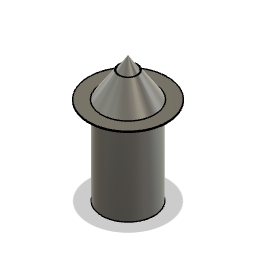
Shielding for CAMECA electrodes v1 (Autodesk Fusion 360 design; units mm, degrees)
Autodesk Fusion 360 part; units mm, degrees
sketch "Sketch1" plane through (0, 0, 0) normal (0, 0, 1) x (1, 0, 0)
  line L0 (0, 3) -> (1, 3) construction
  line L1 (0, 0) -> (3, 0) construction
  line L2 (1, 3) -> (3, 0)
  line L3 (3, 0) -> (4.5, 0)
  line L4 (4.5, 0) -> (4.5, 0.1)
  line L5 (1, 3) -> (1.0832, 3.0555)
  line L6 (4.5, 0.1) -> (3.0535, 0.1)
  line L7 (3.0535, 0.1) -> (1.0832, 3.0555)
  line L8 (0, 4.5) -> (3, 0)
  line L9 (3, 0) -> (3, -10)
  line L10 (3, -10) -> (0, -10)
  line L11 (0, 1.75) -> (0, 22.5)
  line L12 (0, 4.5) -> (0, -10)
  dimension "d1" = 1
  dimension "d3" = 3
  dimension "d4" = 3
  dimension "d5" = 1.5
  dimension "d6" = 0.1
  dimension "d7" = 0.1
  dimension "d9" = 123.69
  dimension "d11" = 10
  constraint horizontal L0
  constraint coincident L1.start origin
  constraint horizontal L1
  constraint parallel L1 L3
  constraint perpendicular L3 L4
  constraint perpendicular L2 L5
  constraint perpendicular L4 L6
  constraint parallel L2 L7
  constraint parallel L2 L8
  constraint vertical L9
  constraint perpendicular L9 L10
  constraint coincident L8.start L11
  constraint perpendicular L10 L12
  measures "d1" distance of L0.start L0.end
  measures "d3" distance of L1.start L1.end
  measures "d4" distance of L1.start L0.start
  measures "d5" distance of L1.end L3.end
  measures "d6" distance of L3.end L4.end
  measures "d7" distance of L0.end L5.end
  measures "d9" angle of L6 L7
  measures "d11" distance of L1.end L9.end
revolve "Revolve1" add sketch "Sketch1" angle 360 about axis through (0, 1.75, 0) along (0, 1, 0) contours L2 L3 L4 L5 L6 L7 L8 makes body 1
revolve "Revolve2" add sketch "Sketch1" angle 360 about axis through (0, 1.75, 0) along (0, 1, 0) separate body contours L2 L8 L9 L10 L11 L12 makes body 2
named bodies: "Shielding", "Shielding Stamp"
